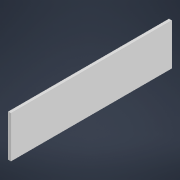
# Autodesk Inventor part: TorraumFrontKlein
Saved by Autodesk Inventor 2021.4 (Build 254397000, 397)
## iProperties
Created: 2022-03-08
Part Number: TorraumFrontKlein
Material: Generic
Document SubType Name: Modeling
Designer: jo_ki
Density: 1 g/cm^3
Appearance: Default
Author: jo_ki
Autodesk Inventor part; units mm, degrees
ref_plane "YZ Plane" through (0, 0, 0) normal (1, 0, 0) x (0, 1, 0)
ref_plane "XZ Plane" through (0, 0, 0) normal (0, 1, 0) x (-1, 0, 0)
ref_plane "XY Plane" through (0, 0, 0) normal (0, 0, 1) x (1, 0, 0)
sketch "Sketch1" plane through (0, 0, 0) normal (1, 0, 0) x (0, 1, 0)
  line L0 (30, 116) -> (-30, 116)
  line L1 (-30, 116) -> (-30, -116)
  line L2 (-30, -116) -> (30, -116)
  line L3 (30, -116) -> (30, 116)
  line L4 (30, 116) -> (-30, -116) construction
  line L5 (-30, 116) -> (30, -116) construction
  point P0 (0, 0)
  dimension "d0" = 232
  dimension "d1" = 60
  constraints: 12 end point, 2 midpoint, 2 parallel, 1 horizontal, 1 perpendicular
  measures "d0" distance between parallel lines of L0 L2
  measures "d1" distance of L1.end L2.end
extrude "Extrusion1" add sketch "Sketch1" along normal blind 4
body "Solid1"
